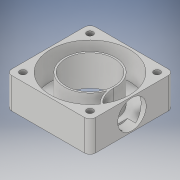
# Autodesk Inventor part: base2
Saved by Autodesk Inventor 2019 (Build 230136000, 136)
## iProperties
Created: 2020-10-29
Part Number: base2
Material: Genérico
Document SubType Name: Modeling
Designer: Juan M. Casillas
Density: 1 g/cm^3
Appearance: Valor por defecto
Author: Juan M. Casillas
Autodesk Inventor part; units mm, degrees
ref_plane "YZ Plane" through (0, 0, 0) normal (1, 0, 0) x (0, 1, 0)
ref_plane "XZ Plane" through (0, 0, 0) normal (0, 1, 0) x (-1, 0, 0)
ref_plane "XY Plane" through (0, 0, 0) normal (0, 0, 1) x (1, 0, 0)
sketch "Sketch1" plane through (0, 0, 0) normal (0, 1, 0) x (-1, 0, 0)
  line L0 (13, 15) -> (-13, 15)
  line L1 (-15, 13) -> (-15, -13)
  line L2 (-13, -15) -> (13, -15)
  line L3 (15, -13) -> (15, 13)
  line L4 (15, 15) -> (-15, -15) construction
  line L5 (-15, 15) -> (15, -15) construction
  circle A0 centre (0, 0) radius 9.15
  circle A1 centre (0, 0) radius 14.13
  arc A2 (15, 13) -> (13, 15) centre (13, 13) ccw
  arc A3 (13, -15) -> (15, -13) centre (13, -13) ccw
  arc A4 (-15, -13) -> (-13, -15) centre (-13, -13) ccw
  arc A5 (-13, 15) -> (-15, 13) centre (-13, 13) ccw
  dimension "d0" = 30
  dimension "d1" = 30
  dimension "d2" = 18.3
  dimension "d3" = 28.26
  dimension "d4" = 2
  constraints: 12 end point, 8 point on circle, 8 point on line, 8 tangent, 6 centre point, 3 equal radius, 2 coincident, 2 midpoint, 2 parallel, 1 horizontal, 1 perpendicular
  measures "d0" distance of L5.end L4.end
  measures "d1" distance of L4.end L5.start
  measures "d2" diameter of A0
  measures "d3" diameter of A1
  measures "d4" radius of A2
extrude "Extrusion1" add sketch "Sketch1" along normal blind 11
sketch "Sketch2" plane through (0, 0, 0) normal (0, -1, 0) x (1, 0, 0)
  line L0 (-15, -13) -> (-15, 13) projected
  arc A0 (-13, 15) -> (-15, 13) centre (-13, 13) ccw projected
  line L1 (-13, 15) -> (13, 15) projected
  arc A1 (15, 13) -> (13, 15) centre (13, 13) ccw projected
  line L2 (15, 13) -> (15, -13) projected
  arc A2 (13, -15) -> (15, -13) centre (13, -13) ccw projected
  line L3 (13, -15) -> (-13, -15) projected
  arc A3 (-15, -13) -> (-13, -15) centre (-13, -13) ccw projected
  point P0 (0, 0)
extrude "Extrusion2" add sketch "Sketch2" against normal blind 1
sketch "Sketch3" plane through (0, 11, 0) normal (0, 1, 0) x (1, 0, 0)
  circle A0 centre (0, 0) radius 9.15 projected
  circle A1 centre (0, 0) radius 8.55
  dimension "d9" = 0.6
  constraints: 1 centre point
  measures "d9" radial gap between concentric circles of A0 A1
extrude "Extrusion3" cut sketch "Sketch3" against normal through all contours A1
sketch "Sketch4" plane through (0, 11, 0) normal (0, 1, 0) x (1, 0, 0)
  circle A0 centre (0, 0) radius 14.13 construction
  line L0 (-13, -15) -> (13, -15) construction
  arc A1 (13, -15) -> (15, -13) centre (13, -13) ccw construction
  line L1 (15, -13) -> (15, 13) construction
  arc A2 (15, 13) -> (13, 15) centre (13, 13) ccw construction
  line L2 (13, 15) -> (-13, 15) construction
  arc A3 (-13, 15) -> (-15, 13) centre (-13, 13) ccw construction
  line L3 (-15, 13) -> (-15, -13) construction
  arc A4 (-15, -13) -> (-13, -15) centre (-13, -13) ccw construction
  line L4 (-12, -12) -> (12, -12) construction
  line L5 (12, -12) -> (12, 12) construction
  line L6 (12, 12) -> (-12, 12) construction
  line L7 (-12, 12) -> (-12, -12) construction
  line L8 (-12, -12) -> (12, 12) construction
  line L9 (12, -12) -> (-12, 12) construction
  point P0 (0, 0)
  dimension "d12" = 24
  dimension "d13" = 24
  constraints: 12 end point, 5 coincident, 3 midpoint, 2 parallel, 1 horizontal, 1 perpendicular
  measures "d12" distance of L6.end L5.end
  measures "d13" distance of L5.end L4.end
hole "Hole1" at (-12, 11, 12) at (-12, 11, -12) at (12, 11, -12) at (12, 11, 12) direction (0, -1, 0) diameter 2.3 depth 10
sketch "Sketch5" plane through (15, 0, -13) normal (1, 0, 0) x (0, 0, -1)
  line L0 (0, 0) -> (0, 11) construction
  line L1 (-26, 11) -> (0, 11) construction
  line L2 (-26, 0) -> (-26, 11) construction
  line L3 (-26, 0) -> (0, 0) construction
  line L4 (-20.5, 10) -> (-5.5, 10)
  line L5 (-5.5, 10) -> (-5.5, 1)
  line L6 (-5.5, 1) -> (-20.5, 1)
  line L7 (-20.5, 1) -> (-20.5, 10)
  line L8 (-20.5, 10) -> (-5.5, 1) construction
  line L9 (-5.5, 10) -> (-20.5, 1) construction
  point P0 (-13, 0)
  point P1 (-13, 5.5)
  dimension "d21" = 15
  dimension "d22" = 9
  constraints: 12 end point, 2 midpoint, 2 parallel, 1 horizontal, 1 perpendicular
  measures "d21" distance of L5.end L6.end
  measures "d22" distance of L4.end L5.end
extrude "Extrusion4" cut sketch "Sketch5" against normal blind 4
sketch "Sketch6" plane through (0, 1, 0) normal (0, 1, 0) x (1, 0, 0)
  line L0 (15, -7.5) -> (11.9753, -7.5) construction
  arc A0 (8.7409, -2.7053) -> (9.1297, -0.6089) centre (0, 0) ccw
  arc A1 (9.1297, -0.6089) -> (11.9753, -7.5) centre (18.8506, -0.6279) ccw
  arc A2 (8.7409, -2.7053) -> (11.6393, -8.0115) centre (18.8506, -0.6279) ccw
  arc A3 (11.6393, -8.0115) -> (11.9753, -7.5) centre (0, 0) ccw
  arc A4 (11.6393, -8.0115) -> (11.9753, -7.5) centre (0, 0) ccw
  dimension "d25" = 0.6
  constraints: 11 point on circle, 6 centre point
  measures "d25" radial gap between concentric circles of A1 A2
extrude "Extrusion5" add sketch "Sketch6" along normal up to surface (10 mm away)
fillet "Fillet1" radius 2 2 edges at (11.9753, 5.5, 7.5) (11.9753, 5.5, -7.5)
sketch "Sketch12" plane through (15, 10, -7.5) normal (0, -1, 0) x (1, 0, 0)
  arc A0 (-2.139, 15) -> (-2.9253, 14.8389) centre (-2.139, 13) ccw projected
  arc A1 (-3.5807, -0.8221) -> (-2.9253, 14.8389) centre (-15, 7.5) ccw projected
  arc A2 (-1.9644, 0) -> (-3.5807, -0.8221) centre (-1.9644, -2) ccw projected
  line L0 (0, 0) -> (-1.9644, 0) projected
  line L1 (0, 15) -> (0, 0) projected
  line L2 (0, 15) -> (-2.139, 15) projected
extrude "Extrusion10" add sketch "Sketch12" along normal up to surface (9 mm away)
sketch "Sketch13" plane through (15, 0, -13) normal (1, 0, 0) x (0, 0, -1)
  line L0 (0, 0) -> (0, 11) construction
  line L1 (-26, 11) -> (0, 11) construction
  line L2 (-26, 0) -> (-26, 11) construction
  line L3 (-26, 0) -> (0, 0) construction
  circle A0 centre (-13, 5.5) radius 5.1
  point P0 (-13, 0)
  dimension "d44" = 10.2
  constraints: 1 centre point
  measures "d44" diameter of A0
extrude "Extrusion11" cut sketch "Sketch13" against normal blind 4
sketch "Sketch8" plane through (20, 0, -13) normal (1, 0, 0) x (0, 0, -1)
  line L0 (-20.5, 10) -> (-5.5, 10) projected
  line L1 (-20.5, 1) -> (-20.5, 10) projected
  line L2 (-5.5, 1) -> (-20.5, 1) projected
  line L3 (-5.5, 10) -> (-5.5, 1) projected
  line L4 (-20.3, 9.8) -> (-5.7, 9.8)
  line L5 (-5.7, 9.8) -> (-5.7, 1.2)
  line L6 (-5.7, 1.2) -> (-20.3, 1.2)
  line L7 (-20.3, 1.2) -> (-20.3, 9.8)
  point P0 (-13, 0)
  dimension "d30" = 0.2
  dimension "d33" = 1
  dimension "d34" = 0.6
  constraints: 16 end point, 6 other
  measures "d33" distance between parallel lines of L1 L4
sketch "Sketch11" plane through (22.6, 0, -13) normal (1, 0, 0) x (0, 0, -1)
  line L0 (-21.3, 10.8) -> (-21.3, 0.2) construction
  line L1 (-21.3, 0.2) -> (-4.7, 0.2) construction
  line L2 (-4.7, 0.2) -> (-4.7, 10.8) construction
  line L3 (-4.7, 10.8) -> (-21.3, 10.8) construction
  circle A0 centre (-13, 5.5) radius 5.125
  point P0 (-13, 0)
  dimension "d39" = 10.25
  constraints: 1 centre point
  measures "d39" diameter of A0
body "Solid1"
